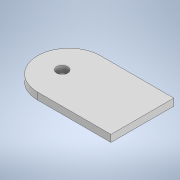
# Autodesk Inventor part: tampa hc 12
Saved by Autodesk Inventor 2022 (Build 260153000, 153)
## iProperties
Created: 2022-04-15
Part Number: tampa hc 12
Material: Genérico
Document SubType Name: Modeling
Designer: Hanter
Density: 1 g/cm^3
Appearance: Padrão
Author: Hanter
Autodesk Inventor part; units mm, degrees
ref_plane "YZ Plane" through (0, 0, 0) normal (1, 0, 0) x (0, 1, 0)
ref_plane "XZ Plane" through (0, 0, 0) normal (0, 1, 0) x (-1, 0, 0)
ref_plane "XY Plane" through (0, 0, 0) normal (0, 0, 1) x (1, 0, 0)
sketch "Esboço1" plane through (0, 0, 0) normal (0, 1, 0) x (-1, 0, 0)
  line L0 (-16, 9) -> (16, 9)
  line L1 (16, 9) -> (16, -9)
  line L2 (16, -9) -> (-16, -9)
  line L3 (-16, -9) -> (-16, 9)
  line L4 (-16, 9) -> (16, -9) construction
  line L5 (8.3086, 4.6736) -> (-16, -9) construction
  arc A0 (16, -9) -> (16, 9) centre (16, 0) ccw
  circle A1 centre (17.962, 0) radius 1.6
  dimension "d2" = 32
  dimension "d3" = 18
  dimension "d5" = 3.2
  dimension "d6" = 1.962
  constraints: 12 end point, 2 centre point, 2 parallel, 2 point on circle, 1 horizontal, 1 midpoint, 1 perpendicular
  measures "d2" distance of L1.end L2.end
  measures "d3" distance of L1.end L0.end
  measures "d5" diameter of A1
  measures "d6" distance from line of L1 A1.centre
extrude "Extrusão1" add sketch "Esboço1" along normal blind 2
sketch "Esboço2" plane through (0, 2, 0) normal (0, 1, 0) x (1, 0, 0)
  line L0 (16, 9) -> (-16, 9) projected
  line L1 (16, 9) -> (5, 9)
  line L2 (5, 9) -> (5, -9)
  line L3 (5, -9) -> (16, -9)
  line L4 (16, -9) -> (16, 9)
  point P0 (0, 0)
  dimension "d9" = 11
  dimension "d10" = 18
  constraints: 8 end point, 2 parallel, 1 horizontal, 1 perpendicular
  measures "d9" distance of L3.end L2.end
  measures "d10" distance of L1.end L2.end
extrude "Extrusão2" cut sketch "Esboço2" against normal blind 2
